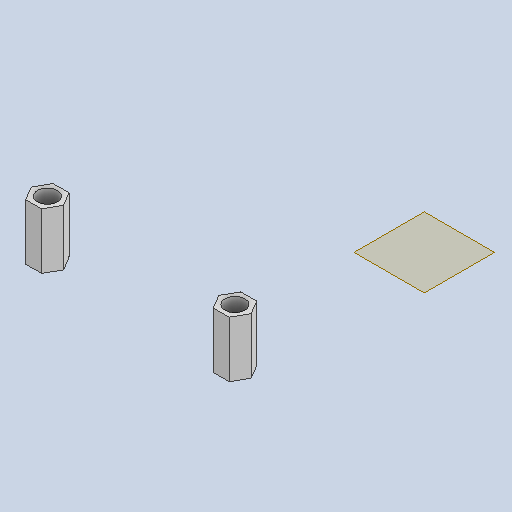
# Autodesk Inventor part: стойка для дисплея
Saved by Autodesk Inventor 2024.2 (Build 282272000, 272)
## iProperties
Created: 2025-12-10
Part Number: стойка для дисплея
Material: Типовые
Document SubType Name: Modeling
Designer: katya_notebook
Density: 1 g/cm^3
Appearance: По умолчанию
Author: katya_notebook
Autodesk Inventor part; units mm, degrees
ref_plane "YZ Plane" through (0, 0, 0) normal (1, 0, 0) x (0, 1, 0)
ref_plane "XZ Plane" through (0, 0, 0) normal (0, 1, 0) x (-1, 0, 0)
ref_plane "РабПлоскость1" through (383.3254, 72.1989, -189.0917) normal (0, 1, 0) x (1, 0, 0)
sketch "Эскиз1" plane through (383.3254, 72.1989, -189.0917) normal (0, 1, 0) x (1, 0, 0)
  circle A0 centre (-6.1976, -17.515) radius 1.3 projected
  circle A1 centre (-29.6976, -17.515) radius 1.3 projected
  circle A2 centre (-29.6976, 6.235) radius 1.3 projected
  circle A3 centre (-6.1976, -17.515) radius 2
  line L0 (-5.2043, -15.779) -> (-4.1976, -17.5072)
  line L1 (-4.1976, -17.5072) -> (-5.1909, -19.2431)
  line L2 (-5.1909, -19.2431) -> (-7.1908, -19.2509)
  line L3 (-7.1908, -19.2509) -> (-8.1976, -17.5227)
  line L4 (-8.1976, -17.5227) -> (-7.2043, -15.7868)
  line L5 (-7.2043, -15.7868) -> (-5.2043, -15.779)
  circle A4 centre (-29.6976, -17.515) radius 2
  line L6 (-28.7236, -15.7682) -> (-27.6978, -17.4851)
  line L7 (-27.6978, -17.4851) -> (-28.6718, -19.2319)
  line L8 (-28.6718, -19.2319) -> (-30.6716, -19.2617)
  line L9 (-30.6716, -19.2617) -> (-31.6974, -17.5448)
  line L10 (-31.6974, -17.5448) -> (-30.7233, -15.798)
  line L11 (-30.7233, -15.798) -> (-28.7236, -15.7682)
  circle A5 centre (-6.1976, -17.515) radius 1.25
  circle A6 centre (-29.6976, -17.515) radius 1.25
  point P0 (-383.3254, -189.0917)
  dimension "d0" = 4
  dimension "d1" = 4
  dimension "d5" = 2.5
  dimension "d6" = 2.5
  constraints: 24 end point, 6 coincident, 2 centre point, 32 other
  measures "d5" diameter of A5
  measures "d6" diameter of A6
ref_plane "РабПлоскость2" through (351.6278, 65.1989, -197.3267) normal (0, 1, 0) x (0, 0, 1)
extrude "Выдавливание1" add sketch "Эскиз1" against normal up to surface (7 mm away) contours A0 | A1 | L1 L2 L3 L4 L5 L0 | L7 L8 L9 L10 L11 L6
